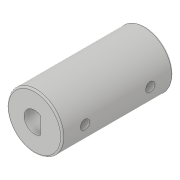
# Autodesk Inventor part: schroefkoppeling motor en overbrening
Saved by Autodesk Inventor 2019 (Build 230136000, 136)
## iProperties
Created: 2020-03-11
Part Number: schroefkoppeling motor en overbrening
Material: Generic
Document SubType Name: Modeling
Designer: stef_
Density: 1 g/cm^3
Appearance: Default
Author: stef_
Autodesk Inventor part; units mm, degrees
ref_plane "YZ Plane" through (0, 0, 0) normal (1, 0, 0) x (0, 1, 0)
ref_plane "XZ Plane" through (0, 0, 0) normal (0, 1, 0) x (-1, 0, 0)
sketch "Sketch1" plane through (0, 0, 0) normal (0, 0, 1) x (1, 0, 0)
  circle A0 centre (0, 0) radius 8.5
  circle A1 centre (0, 0) radius 3.69
  dimension "d0" = 17
  dimension "d3" = 7.38
  dimension "d20" = 4.81
  constraints: 2 centre point, 2 coincident
  measures "d0" diameter of A0
  measures "d3" diameter of A1
  measures "d20" radial gap between concentric circles of A0 A1
extrude "Extrusion2" add sketch "Sketch1" along normal blind 18
sketch "Sketch2" plane through (0, 0, 18) normal (0, 0, 1) x (1, 0, 0)
  circle A0 centre (0, 0) radius 8.5
  circle A1 centre (0, 0) radius 8.5 projected
  constraints: 1 centre point, 1 coincident, 1 concentric
extrude "Extrusion3" add sketch "Sketch2" along normal blind 4
sketch "Sketch3" plane through (0, 0, 22) normal (0, 0, 1) x (1, 0, 0)
  arc A0 (1.815, 2.6173) -> (1.815, -2.6173) centre (0, 0) ccw
  circle A1 centre (0, 0) radius 8.5
  line L0 (1.815, 2.6173) -> (1.815, -2.6173)
  circle A2 centre (0, 0) radius 8.5 projected
  dimension "d8" = 6.37
  dimension "d11" = 5
  dimension "d12" = 1.815
  constraints: 2 centre point, 2 coincident, 2 end point, 2 point on circle, 1 concentric, 1 vertical
  measures "d8" diameter of A0
  measures "d12" distance from line of L0 point (0, 0)
extrude "Extrusion4" add sketch "Sketch3" along normal blind 12
ref_plane "Work Plane2" through (6, -1.3086, 34) normal (1, 0, 0) x (0, -1, 0)
ref_plane "Work Plane1" through (1.815, -1.3086, 34) normal (1, 0, 0) x (0, -1, 0)
sketch "Sketch4" plane through (6, -1.3086, 34) normal (1, 0, 0) x (0, -1, 0)
  circle A0 centre (-1.3086, 7) radius 1.425
  circle A1 centre (-1.3086, 27) radius 1.425
  line L0 (-9.8086, 0) -> (7.1914, 0) projected
  line L1 (7.1914, 34) -> (-9.8086, 34) projected
  point P0 (-1.3086, 34)
  dimension "d14" = 2.85
  dimension "d15" = 7
  dimension "d16" = 7
  constraints: 2 centre point, 1 equal radius
  measures "d14" diameter of A0
  measures "d15" distance from line of L0 A0.centre
  measures "d16" distance from line of L1 A1.centre
extrude "Extrusion5" cut sketch "Sketch4" along normal blind 6.185 and the other way blind 5
fillet "Fillet1" radius 0.5 2 edges at (-8.5, 0, 34) (-8.5, 0, 0)
body "Solid2"
